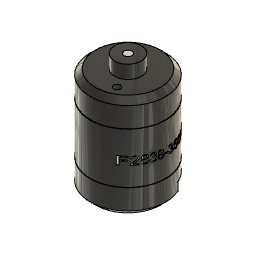
Moteur-F2838-350KV_KOSMOS3-0 (Autodesk Fusion 360 design; units mm, degrees)
Autodesk Fusion 360 part; units mm, degrees
sketch "Esquisse1" plane through (0, 0, 0) normal (0, 0, 1) x (1, 0, 0)
  circle A0 centre (0, 0) radius 14.2
  circle A1 centre (0, 0) radius 1.5
  dimension "d1" = 28.4
  dimension "d2" = 3
  constraint coincident A0.centre A1.centre
  measures "d1" diameter of A0
  measures "d2" diameter of A1
extrude "Extrusion1" add sketch "Esquisse1" along normal blind 9.6 makes body 1
sketch "Esquisse2" plane through (0, 0, 0) normal (0, 0, -1) x (1, 0, 0)
  circle A0 centre (0, 0) radius 1.5
  circle A1 centre (0, 0) radius 14.2
  circle A2 centre (-3.9599, 8.082) radius 1.25
  circle A3 centre (3.9599, -8.082) radius 1.25
  dimension "d6" = 2.5
  dimension "d7" = 2.5
  measures "d6" diameter of A2
  measures "d7" diameter of A3
extrude "Extrusion2" cut sketch "Esquisse2" against normal blind 7.5 contours A2 | A3 bodies 1
chamfer "Chanfrein1" distance 2 angle 45 1 edges at (-13.239, -5.1349, 0) on bodies 1
move_body "Déplacer1" bodies 1 to x (1, 0, 0) y (0, 1, 0) z (0, 0, 1) at (-130, 100, 0)
sketch "Esquisse3" plane through (0, 0, 0) normal (0, 0, 1) x (1, 0, 0)
  circle A0 centre (0, 0) radius 14.2
  circle A1 centre (0, 0) radius 1.5
  circle A2 centre (0.0017, -9) radius 1.25
  circle A3 centre (-0.0017, 9) radius 1.25
  circle A4 centre (-9, -0.0012) radius 1.25
  circle A5 centre (9, 0.0022) radius 1.25
  line L0 (10.0433, -10.0385) -> (5.7997, -5.7969)
  line L1 (5.7997, -5.7969) -> (9.3344, -2.2605)
  line L2 (5.7997, -5.7969) -> (2.265, -9.3333)
  line L3 (3.3254, -8.2724) -> (9.3344, -2.2605)
  line L4 (3.3259, -10.3937) -> (5.8654, -12.932)
  line L5 (8.2739, -3.3214) -> (7.114, -4.4819)
  line L6 (10.3953, -3.3209) -> (12.9348, -5.8592)
  arc A6 (3.3254, -8.2724) -> (3.3259, -10.3937) centre (4.3863, -9.3328) ccw
  arc A7 (10.3953, -3.3209) -> (8.2739, -3.3214) centre (9.3349, -4.3818) ccw
  dimension "d12" = 3
  dimension "d14" = 2.5
  dimension "d15" = 2.5
  dimension "d16" = 2.5
  dimension "d17" = 2.5
  dimension "d19" = 6
  dimension "d23" = 1.5
  dimension "d24" = 1.5
  constraint coincident A0.centre A1.centre
  constraint coincident A0 L4.end
  constraint perpendicular L2 L4
  constraint coincident L1 L5.end
  constraint perpendicular L4 L5
  constraint coincident A0 L6.end
  constraint coincident L2.end L4
  constraint coincident L2.end L3
  constraint tangent L4 A6
  constraint tangent L3 A6
  constraint coincident L1.end L6
  constraint tangent L5 A7
  constraint tangent L6 A7
  measures "d12" diameter of A1
  measures "d14" diameter of A2
  measures "d15" diameter of A3
  measures "d16" diameter of A4
  measures "d17" diameter of A5
  measures "d19" distance of L0.start L0.end
  measures "d23" radius of A6
  measures "d24" radius of A7
extrude "Extrusion3" add sketch "Esquisse3" along normal blind 9.6 separate body contours A0 L1 L2 L3 L4 L5 L6 A6 A7 | A0 L0 L2 L3 L4 A6 | A0 L0 L1 L3 L5 L6 A7 | A2 | A3 | A4 | A5 makes body 2
sketch "Esquisse4" plane through (0, 0, 0) normal (0, 0, -1) x (1, 0, 0)
  circle A0 centre (0, 0) radius 1.5
  circle A1 centre (0, 0) radius 14.2
  circle A2 centre (-0.0017, 9) radius 1.25
  circle A3 centre (9, 0.0022) radius 1.25
  circle A4 centre (0, 0) radius 14.2
  circle A5 centre (0, 0) radius 1.5
  circle A6 centre (-9, -0.0012) radius 1.25
  circle A7 centre (0.0017, -9) radius 1.25
  arc A8 (10.3953, -3.3209) -> (8.2739, -3.3214) centre (9.3349, -4.3818) ccw
  arc A9 (3.3254, -8.2724) -> (3.3259, -10.3937) centre (4.3863, -9.3328) ccw
  line L0 (8.2739, -3.3214) -> (7.114, -4.4819)
  line L1 (10.3953, -3.3209) -> (12.9348, -5.8592)
  line L2 (3.3259, -10.3937) -> (5.8654, -12.932)
  line L3 (3.3254, -8.2724) -> (7.114, -4.4819)
  constraint tangent A9 L3
extrude "Extrusion5" cut sketch "Esquisse4" against normal blind 4.5 contours A2 | A3 | A6 | A7 bodies 2
extrude "Extrusion4" cut sketch "Esquisse4" against normal blind 4.9 contours A1 A4 A8 A9 L0 L1 L2 L3 picked at (6.5783, -7.8297) bodies 2
chamfer "Chanfrein2" distance 2 angle 45 1 edges at (-10.0433, -10.0385, 0) on bodies 2
move_body "Déplacer2" bodies 2 to x (1, 0, 0) y (0, 1, 0) z (0, 0, 1) at (-90, 60, 0)
sketch "Esquisse5" plane through (0, 0, 0) normal (0, 0, 1) x (1, 0, 0)
  circle A0 centre (0, 0) radius 14.2
  circle A1 centre (0, 0) radius 1.5
  dimension "d32" = 28.4
  dimension "d33" = 3
  constraint coincident A0.centre A1.centre
  measures "d32" diameter of A0
  measures "d33" diameter of A1
extrude "Extrusion6" add sketch "Esquisse5" along normal blind 19.2 separate body makes body 3
chamfer "Chanfrein3" distance 0.1 angle 45 1 edges at (-13.239, -5.1349, 0) on bodies 3
chamfer "Chanfrein4" distance 0.1 angle 45 1 edges at (-13.239, -5.1349, 19.2) on bodies 3
move_body "Déplacer3" bodies 3 to x (1, 0, 0) y (0, 1, 0) z (0, 0, 1) at (-120, 45, 0)
sketch "Esquisse6" plane through (0, 0, 0) normal (0, 0, 1) x (1, 0, 0)
  circle A0 centre (0, 0) radius 1.5
  dimension "d38" = 3
  measures "d38" diameter of A0
extrude "Extrusion7" add sketch "Esquisse6" against normal blind 48.7 separate body makes body 4
move_body "Déplacer4" bodies 4 to x (1, 0, 0) y (0, 1, 0) z (0, 0, 1) at (-65, 0, 50)
copy_body "Corps->Comp1" bodies 4 removing the originals makes body 5 in component "Component"
copy_body "Corps->Comp2" bodies 1 removing the originals makes body 6 in component "Component'"
move_body "Déplacer5" bodies 3 to x (1, 0, 0) y (0, 1, 0) z (0, 0, 1) at (0, -30, 0)
copy_body "Corps->Comp3" bodies 3 removing the originals makes body 7 in component "Component''"
copy_body "Corps->Comp4" bodies 2 removing the originals makes body 8 in component "Component'''"
move_body "Déplacer1'" bodies 6 to x (-1, 0, 0) y (0, 1, 0) z (0, 0, -1) at (-252.0801, 0, 15) in component "Component'"
sketch "Esquisse7" plane through (0, 0, 44.7) normal (0, 0, 1) x (-1, 0, 0)
  circle A0 centre (65, 0) radius 1.5
  circle A1 centre (68.9599, -8.082) radius 1.25
  circle A2 centre (61.0401, 8.082) radius 1.25
  circle A3 centre (65, 0) radius 12.2
  circle A4 centre (65, 0) radius 5
  dimension "d53" = 10
  constraint concentric A0 A4
  measures "d53" diameter of A4
extrude "Extrusion1'" add sketch "Esquisse7" along normal blind 5 contours A4 sketch seen with x (1, 0, 0) y (0, 1, 0) z (0, 0, 1) at (-57.0801, 100, -29.7) bodies 6 in component "Component'"
sketch "Esquisse8" plane through (0, 0, 0) normal (0, 0, 1) x (1, 0, 0)
  circle A0 centre (0, 0) radius 5
  circle A1 centre (0, 0) radius 1.5
  dimension "d56" = 10
  dimension "d57" = 3
  constraint coincident A0.centre A1.centre
  measures "d56" diameter of A0
  measures "d57" diameter of A1
extrude "Extrusion8" add sketch "Esquisse8" along normal blind 5 separate body makes body 9
chamfer "Chanfrein5" distance 0.5 distance2 2.7 1 edges at (-4.6616, -1.8081, 0) measured on face at (4.9938, -0.2492, 3.3333) on bodies 9
chamfer "Chanfrein6" distance 2.7 distance2 0.5 1 edges at (-4.6616, -1.8081, 5) measured on face at (3.8091, -0.3229, 5) on bodies 9
move_body "Déplacer6" bodies 9 to x (1, 0, 0) y (0, 1, 0) z (0, 0, 1) at (-20, 0, 0)
copy_body "Corps->Comp5" bodies 9 removing the originals makes body 10 in component "Component''''"
move_body "Déplacer1''" bodies 5 to x (1, 0, 0) y (0, 1, 0) z (0, 0, 1) at (0, 0, -0.3) in component "Component"
sketch "Esquisse9" plane through (0, 0, 0) normal (1, 0, 0) x (0, 1, 0)
ref_plane "Plan de construction1" through (-50.8, 0, 26.9604) normal (1, 0, 0) x (0, -1, 0)
sketch "Esquisse10" plane through (-50.8, 0, 26.9604) normal (1, 0, 0) x (0, 1, 0)
ref_plane "Plan de construction2" through (-50.8, 0, 25.2012) normal (1, 0, 0) x (0, -1, 0)
sketch "Esquisse11" plane through (-50.8, 0, 25.2012) normal (1, 0, 0) x (0, 1, 0)
  line L0 (-12, -5) -> (12, -5) construction
  line L1 (12, -5) -> (12, 4) construction
  line L2 (12, 4) -> (-12, 4) construction
  line L3 (-12, 4) -> (-12, -5) construction
  text T0 "F2838-350KV" font "Arial" height 3 align left middle in box 24 x 9 at (-12, -5) x (1, 0) y (0, 1) spacing 1
extrude "Extrusion1''" add sketch "Esquisse11" along normal blind 0.01 from the near side of the face at (-105.8177, 14.2922, 12.7667) text T0 sketch seen with x (1, 0, 0) y (0, 1, 0) z (0, 0, 1) at (-55, 15, -15.9) on bodies 7 bodies 7 in component "Component''"
ref_plane "Plan de construction3" through (-67.5, 4.3301, 47.3743) normal (-0.5, 0.866025, 0) x (0.866025, 0.5, 0)
sketch "Esquisse12" plane through (-67.5, 4.3301, 47.3743) normal (-0.5, 0.866025, 0) x (0.866025, 0.5, 0)
  circle A0 centre (0, 0) radius 1.3
  dimension "d73" = 2.6
  constraint coincident A0.centre origin
  measures "d73" diameter of A0
extrude "Extrusion2'" cut sketch "Esquisse12" against normal blind 0.8 from the near side of the face at (-127.0739, 100.2492, 18.3333) sketch seen with x (1, 0, 0) y (0, 1, 0) z (0, 0, 1) at (-57.0801, 100, -29.7) on bodies 6 bodies 6 in component "Component'"
ref_plane "Plan de construction4" through (-65, 5, 3.0595) normal (0, 1, 0) x (1, 0, 0)
sketch "Esquisse13" plane through (-65, 5, 3.0595) normal (0, 1, 0) x (1, 0, 0)
  circle A0 centre (0, -1) radius 1.3
  dimension "d77" = 2.6
  measures "d77" diameter of A0
extrude "Extrusion1'''" cut sketch "Esquisse13" against normal blind 0.8 from the near side of the face at (-15.0062, -0.2492, 3.1667) sketch seen with x (1, 0, 0) y (0, 1, 0) z (0, 0, 1) at (45, 0, -1.3) on bodies 10 bodies 10 in component "Component''''"
extrude "Extrusion1''''" cut 1 faces at (-82.5539, 66.9614, 4.9) along direction (0, 0, 1) blind 1.4 on bodies 8 bodies 8 in component "Component'''"
extrude "Extrusion2''" cut 1 faces at (-82.5539, 66.9614, 6.3) along direction (0, 0, 1) blind 0.1 on bodies 8 bodies 8 in component "Component'''"
extrude "Extrusion3'" add 1 faces at (-82.5539, 66.9614, 6.4) along direction (0, 0, -1) blind 1.4 on bodies 8 bodies 8 in component "Component'''"
component "Component" placed x (1, 0, 0) y (0, 1, 0) z (0, 0, 1) at (0, 0, 0)
component "Component'" placed x (1, 0, 0) y (0, 1, 0) z (0, 0, 1) at (57.0801, -100, 29.7)
component "Component''" placed x (1, 0, 0) y (0, 1, 0) z (0, 0, 1) at (55, -15, 15.9)
component "Component'''" placed x (1, 0, 0) y (0, 1, 0) z (0, 0, 1) at (25, -60, 6.3)
component "Component''''" placed x (1, 0, 0) y (0, 1, 0) z (0, 0, 1) at (-45, 0, 1.3)
